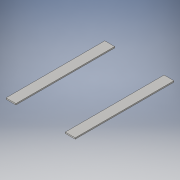
# Autodesk Inventor part: Part9
Saved by Autodesk Inventor 2016 (Build 200138000, 138)
## iProperties
Created: 2016-01-16
Part Number: Part9
Material: Generic
Document SubType Name: Modeling
Designer: Thariq
Density: 1 g/cm^3
Appearance: Default
Author: Thariq
Autodesk Inventor part; units mm, degrees
ref_plane "YZ Plane" through (0, 0, 0) normal (1, 0, 0) x (0, 1, 0)
ref_plane "XZ Plane" through (0, 0, 0) normal (0, 1, 0) x (-1, 0, 0)
ref_plane "XY Plane" through (0, 0, 0) normal (0, 0, 1) x (1, 0, 0)
sketch "Sketch1" plane through (0, 0, 0) normal (0, 1, 0) x (-1, 0, 0)
  line L0 (0, 0) -> (25.4, 0)
  line L1 (25.4, 0) -> (25.4, -254)
  line L2 (25.4, -254) -> (0, -254)
  line L3 (0, -254) -> (0, 0)
  line L4 (-127, 0) -> (-152.4, 0)
  line L5 (-152.4, 0) -> (-152.4, -254)
  line L6 (-152.4, -254) -> (-127, -254)
  line L7 (-127, -254) -> (-127, 0)
  dimension "d0" = 25.4
  dimension "d1" = 25.4
  dimension "d2" = 127
  dimension "d3" = 254
  constraints: 16 end point, 4 parallel, 2 horizontal, 2 perpendicular, 2 point on line
  measures "d0" distance between parallel lines of L1 L3
  measures "d1" distance between parallel lines of L7 L5
  measures "d2" distance between parallel lines of L3 L7
  measures "d3" distance between parallel lines of L4 L6
extrude "Extrusion1" add sketch "Sketch1" along normal blind 3.175
body "Solid1"
